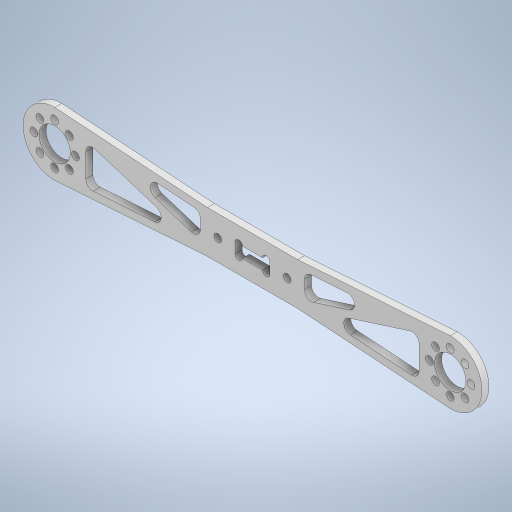
# Autodesk Inventor part: 腕
Saved by Autodesk Inventor 2024 (Build 280153000, 153)
## iProperties
Created: 2023-03-29
Part Number: 腕
Material: アルミニウム 2014-T4
Document SubType Name: Modeling
Designer: right
Density: 2.8 g/cm^3
Appearance: サテン
Mass: 6.80799 g
Surface Area: 37.95 cm^2
Volume: 2.43142 cm^3
Author: right
Autodesk Inventor part; units mm, degrees
ref_plane "YZ Plane" through (0, 0, 0) normal (1, 0, 0) x (0, 1, 0)
ref_plane "XZ Plane" through (0, 0, 0) normal (0, 1, 0) x (-1, 0, 0)
ref_plane "XY Plane" through (0, 0, 0) normal (0, 0, 1) x (1, 0, 0)
sketch "スケッチ1" plane through (0, 0, 0) normal (0, 0, 1) x (1, 0, 0)
  circle A0 centre (0, 0) radius 4.5
  circle A1 centre (0, 0) radius 6 construction
  circle A2 centre (0, 6) radius 1.1
  circle A3 centre (-4.2426, 4.2426) radius 1.1
  circle A4 centre (-6, 0) radius 1.1
  circle A5 centre (-4.2426, -4.2426) radius 1.1
  circle A6 centre (0, -6) radius 1.1
  circle A7 centre (4.2426, -4.2426) radius 1.1
  circle A8 centre (6, 0) radius 1.1
  circle A9 centre (4.2426, 4.2426) radius 1.1
  circle A10 centre (0, 0) radius 9.1
  line L0 (0, 9.1) -> (114, 9.1)
  line L1 (114, 9.1) -> (114, -9.1)
  line L2 (114, -9.1) -> (0, -9.1)
  line L3 (0, -9.1) -> (0, 9.1) construction
  line L4 (57, 9.1) -> (57, -9.1) construction
  circle A11 centre (114, 0) radius 4.5
  circle A12 centre (114, 0) radius 6 construction
  circle A13 centre (114, 6) radius 1.1
  circle A14 centre (118.2426, 4.2426) radius 1.1
  circle A15 centre (120, 0) radius 1.1
  circle A16 centre (118.2426, -4.2426) radius 1.1
  circle A17 centre (114, -6) radius 1.1
  circle A18 centre (109.7574, -4.2426) radius 1.1
  circle A19 centre (108, 0) radius 1.1
  circle A20 centre (109.7574, 4.2426) radius 1.1
  circle A21 centre (114, 0) radius 9.1
  line L5 (114, -9.1) -> (114, 9.1) construction
  point P0 (0, 0)
  point P1 (0, -9.1)
  point P2 (114, -9.1)
  dimension "d1" = 12
  dimension "d0" = 9
  dimension "d2" = 2.2
  dimension "d5" = 360
  dimension "d7" = 2
  dimension "d8" = 57
  constraints: 18 centre point, 12 end point, 12 symmetric about line, 6 coincident, 3 horizontal, 3 midpoint, 3 vertical alignment, 2 parallel, 2 vertical, 1 perpendicular, 36 other
  measures "d0" diameter of A0
  measures "d2" diameter of A2
  measures "d8" distance from line of point (0, 0) L4
extrude "押し出し1" add sketch "スケッチ1" along normal blind 2 contours A10 | A10 L0 A21 L2 | A21 L1 A17 A11 A13 | L1 A13 A11 A17 A21
sketch "スケッチ2" plane through (0, 0, 2) normal (0, 0, 1) x (1, 0, 0)
  line L0 (52, -1.5) -> (62, -1.5)
  line L1 (62, -1.5) -> (62, 1.5)
  line L2 (62, 1.5) -> (52, 1.5)
  line L3 (52, 1.5) -> (52, -1.5)
  line L4 (114, 9.1) -> (0, 9.1) projected
  circle A0 centre (53.05, 1.5) radius 1.05
  line L5 (52, 0) -> (62, 0) construction
  line L6 (57, 1.5) -> (57, -1.5) construction
  circle A1 centre (60.95, 1.5) radius 1.05
  circle A2 centre (53.05, -1.5) radius 1.05
  circle A3 centre (60.95, -1.5) radius 1.05
  circle A4 centre (47, 0) radius 1.1
  circle A5 centre (67, 0) radius 1.1
  point P0 (0, 0)
  point P1 (57, 9.1)
  point P2 (59.9, 1.5)
  point P3 (54.1, 1.5)
  point P4 (54.1, -1.5)
  point P5 (59.9, -1.5)
  point P6 (62, -1.5)
  point P7 (62, 1.5)
  dimension "d13" = 2.1
  dimension "d11" = 10
  dimension "d12" = 3
  dimension "d14" = 2.2
  dimension "d15" = 5
  constraints: 12 end point, 5 midpoint, 4 centre point, 4 symmetric about line, 2 horizontal, 2 horizontal alignment, 2 parallel, 1 perpendicular, 1 point on line, 1 vertical alignment, 9 other
  measures "d11" distance of L2.end L1.end
  measures "d12" distance of L1.end L0.end
  measures "d14" diameter of A4
  measures "d15" distance of L5.start A4.centre
extrude "押し出し2" cut sketch "スケッチ2" against normal blind 10
sketch "スケッチ3" plane through (0, 0, 0) normal (0, 0, -1) x (-1, 0, 0)
  line L0 (-70, -6.1) -> (-44, -6.1)
  line L1 (-44, -6.1) -> (-44, 6.1)
  line L2 (-44, 6.1) -> (-70, 6.1)
  line L3 (-70, 6.1) -> (-70, -6.1)
  line L4 (-59.9, 1.5) -> (-54.1, 1.5) projected
  circle A0 centre (-67, 0) radius 1.1 projected
  line L5 (-54.1, -1.5) -> (-59.9, -1.5) projected
  line L6 (0, -9.1) -> (-114, -9.1) projected
  line L7 (-70, -6.1) -> (-114, -9.1)
  line L8 (-70, 0) -> (-120, 0) construction
  line L9 (-57, 6.1) -> (-57, 9.1) construction
  line L10 (-114, 9.1) -> (0, 9.1) projected
  line L11 (-70, 6.1) -> (-114, 9.1)
  line L12 (-114, -9.1) -> (0, -9.1)
  line L13 (-44, -6.1) -> (0, -9.1)
  line L14 (-44, 6.1) -> (0, 9.1)
  point P0 (0, 0)
  point P1 (-57, 1.5)
  point P2 (-57, 1.5)
  point P3 (-57, -6.1)
  point P4 (-57, -1.5)
  point P5 (0, 9.1)
  point P6 (-114, 9.1)
  dimension "d18" = 3
  dimension "d29" = 3
  dimension "d31" = 3
  constraints: 22 end point, 7 midpoint, 4 symmetric about line, 2 horizontal, 2 parallel, 1 perpendicular, 1 vertical alignment
  measures "d18" distance from line of L3 A0.centre
  measures "d29" distance from line of L10 L9.start
  measures "d31" distance between parallel lines of L6 L0
extrude "押し出し3" cut sketch "スケッチ3" against normal blind 10 contours L0 L13 L6 L7 | L11 L10 L14 L2
sketch "スケッチ4" plane through (0, 0, 0) normal (0, 0, -1) x (-1, 0, 0)
  line L0 (-9, 4.1405) -> (-9, -6.3815)
  line L1 (-9, -6.3815) -> (-42, -4.1315)
  line L2 (-44, -6.1) -> (0, -9.1) projected
  line L3 (-52, 1.5) -> (-52, -1.5) projected
  circle A0 centre (-6, 0) radius 1.1 projected
  line L4 (-9, 0) -> (-26.6492, 0) construction
  circle A1 centre (-47, 0) radius 1.1 construction
  line L5 (-70, -6.1) -> (-44, -6.1) construction
  line L6 (-57, -6.1) -> (-57, 6.1) construction
  line L7 (-44, 6.1) -> (-70, 6.1) construction
  line L8 (-9, -4.1405) -> (-9, 6.3815)
  line L9 (-9, 6.3815) -> (-42, 4.1315)
  line L10 (-42, 4.1315) -> (-42, -4.1315)
  line L11 (0, 9.1) -> (-44, 6.1) construction
  line L12 (-105, 4.1405) -> (-105, -6.3815)
  line L13 (-105, -6.3815) -> (-72, -4.1315)
  line L14 (-105, 0) -> (-87.3508, 0) construction
  line L15 (-105, 6.3815) -> (-72, 4.1315)
  line L16 (-105, -4.1405) -> (-105, 6.3815)
  line L17 (-72, 4.1315) -> (-72, -4.1315)
  line L18 (-105, 6.3815) -> (-72, -4.1315)
  line L19 (-72.0515, -5.1646) -> (-105.5556, 5.509)
  line L20 (-105.5556, 5.509) -> (-104.9485, 7.4146)
  line L21 (-104.9485, 7.4146) -> (-71.4444, -3.259)
  line L22 (-71.4444, -3.259) -> (-72.0515, -5.1646)
  line L23 (-72.0515, -5.1646) -> (-104.9485, 7.4146) construction
  line L24 (-105.5556, 5.509) -> (-71.4444, -3.259) construction
  line L25 (-41.9485, -5.1646) -> (-8.4444, 5.509)
  line L26 (-9.0515, 7.4146) -> (-42.5556, -3.259)
  point P0 (0, 0)
  point P1 (-105, -4.1405)
  point P2 (-88.5, 1.125)
  point P3 (-42, -3.082)
  point P4 (-13.1915, 6.0957)
  point P5 (-9, 5.332)
  point P6 (-39.2864, -4.3165)
  point P7 (-100.8085, 6.0957)
  point P8 (-72, -3.082)
  point P9 (-74.7136, -4.3165)
  point P10 (-105, 5.332)
  dimension "d23" = 3
  dimension "d24" = 2.1
  dimension "d25" = 5
  dimension "d30" = 2
  constraints: 44 end point, 15 symmetric about line, 6 parallel, 5 midpoint, 2 point on line, 2 vertical, 1 horizontal, 1 horizontal alignment, 1 perpendicular
  measures "d23" distance from line of A0.centre L0
  measures "d24" distance between parallel lines of L2 L1
  measures "d25" horizontal distance of L1.end A1.centre
  measures "d30" distance of L19.end L20.end
extrude "押し出し4" cut sketch "スケッチ4" against normal through all contours L0 L1 L25 L8 | L26 L10 L9 | L16 L19 L13 L12 | L15 L17 L21
fillet "フィレット1" radius 2 12 edges at (72, 4.1315, 1) (105, -6.3815, 1) (9, -6.3815, 1) (42, 4.1315, 1) (74.7136, -4.3165, 1) (72, -3.082, 1) (100.8085, 6.0957, 1) (39.2864, -4.3165, 1) (42, -3.082, 1) (13.1915, 6.0957, 1) (9, 5.332, 1) (105, 5.332, 1)
equation "\"d31\" = d29"
